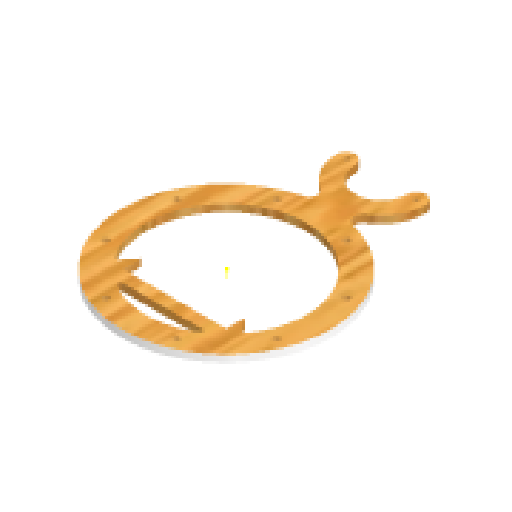
# Autodesk Inventor part: SparRing Curved
Saved by Autodesk Inventor 2025.2 (Build 292293000, 293)
## iProperties
Created: 2024-11-15
Part Number: SparRing Curved
Material: Plywood, Finish
Document SubType Name: Modeling
Designer: alexb
Density: 0.552 g/cm^3
Appearance: Plywood - New
Finish1_Area: 30458.089 mm^2
Finish1_Appearance: Plywood - New
Author: alexb
Autodesk Inventor part; units mm, degrees
ref_plane "YZ Plane" through (0, 0, 0) normal (1, 0, 0) x (0, 1, 0)
ref_plane "XZ Plane" through (0, 0, 0) normal (0, 1, 0) x (-1, 0, 0)
ref_plane "XY Plane" through (0, 0, 0) normal (0, 0, 1) x (1, 0, 0)
sketch "Sketch1" plane through (0, 0, 0) normal (0, 1, 0) x (-1, 0, 0)
  arc A0 (20, -82.6136) -> (-20, -82.6136) centre (0, 0) ccw
  line L0 (0, 0) -> (0, -85)
  line L1 (0, 0) -> (32.5281, -78.5298)
  circle A1 centre (0, 0) radius 75 construction
  circle A2 centre (28.7013, -69.291) radius 2.5
  line L2 (41, -41) -> (-41, -41) construction
  line L3 (-41, -41) -> (-41, 41) construction
  line L4 (-41, 41) -> (41, 41) construction
  line L5 (41, 41) -> (41, -41) construction
  line L6 (0, 0) -> (-85, 0)
  circle A3 centre (69.291, -28.7013) radius 2.5
  circle A4 centre (69.291, 28.7013) radius 2.5
  circle A5 centre (28.7013, 69.291) radius 2.5
  circle A6 centre (-28.7013, 69.291) radius 2.5
  circle A7 centre (-69.291, 28.7013) radius 2.5
  circle A8 centre (-69.291, -28.7013) radius 2.5
  circle A9 centre (-28.7013, -69.291) radius 2.5
  line L7 (42, 27) -> (42, 42)
  line L8 (42, 42) -> (-42, 42)
  line L9 (-42, 42) -> (-42, 27)
  line L10 (42, 27) -> (52.0326, 38.9564)
  line L11 (-39, 52) -> (39, 52)
  line L12 (-42, 27) -> (-52.0326, 38.9564)
  arc A10 (-52.0326, 38.9564) -> (52.0326, 38.9564) centre (0, 0) ccw
  arc A11 (39, 52) -> (-39, 52) centre (0, 0) ccw
  arc A12 (21, -126) -> (-21, -126) centre (0, -126) ccw
  line L13 (0, -105) -> (0, -85) construction
  arc A13 (-20, -82.6136) -> (20, -82.6136) centre (0, 0) ccw construction
  line L14 (0, -126) -> (36, -126) construction
  arc A14 (27.5132, -133.4348) -> (-27.5132, -133.4348) centre (0, -126) ccw
  circle A15 centre (28.5, -126) radius 2
  circle A16 centre (-28.5, -126) radius 2
  arc A17 (-20, -96.0667) -> (-36, -126) centre (0, -126) ccw
  arc A18 (36, -126) -> (20, -96.0667) centre (0, -126) ccw
  arc A19 (21, -126) -> (36, -126) centre (28.5, -126) ccw
  line L15 (0, -126) -> (-36, -126) construction
  arc A20 (-36, -126) -> (-21, -126) centre (-28.5, -126) ccw
  line L16 (-20, -89.3401) -> (-15, -89.3401) construction
  spline S0 degree 4 poles (-20, -82.6136) (-15.4558, -83.7137) (-12.0866, -90.2039) (-16.4143, -93.671) (-20, -96.0667) knots 0 0 0 0 0 1 1 1 1 1
  spline S1 degree 4 poles (20, -82.6136) (15.4558, -83.7137) (12.0866, -90.2039) (16.4143, -93.671) (20, -96.0667) knots 0 0 0 0 0 1 1 1 1 1
  line L17 (20, -89.3401) -> (15, -89.3401) construction
  line L18 (20, -96.0667) -> (20, -82.6136) construction
  line L19 (-20, -96.0667) -> (-20, -82.6136) construction
  point P0 (0, -41)
  point P1 (-41, 0)
  point P2 (0, 52)
  point P3 (17.5, -89.3401)
  dimension "d4" = 150
  dimension "d0" = 170
  dimension "d3" = 22.5
  dimension "d6" = 82
  dimension "d10" = 360
  dimension "d12" = 5
  dimension "d13" = 1
  dimension "d14" = 1
  dimension "d15" = 1
  dimension "d16" = 15
  dimension "d17" = 40
  dimension "d18" = 10
  dimension "d19" = 40
  dimension "d20" = 20
  dimension "d21" = 42
  dimension "d25" = 20
  dimension "d28" = 57
  dimension "d32" = 360
  dimension "d34" = 4
  dimension "d37" = 15
  dimension "d41" = 5
  dimension "d42" = 6.7266
  dimension "d43" = 6.7266
  dimension "d44" = 30
  constraints: 40 end point, 25 point on circle, 20 centre point, 8 coincident, 8 horizontal, 5 point on line, 5 vertical, 4 midpoint, 3 parallel, 3 perpendicular, 2 concentric, 2 equal length, 1 symmetric about line, 36 other
  measures "d0" diameter of A0
  measures "d3" angle of L0 L1
  measures "d6" distance of L2.start L2.end
  measures "d12" diameter of A9
  measures "d13" distance between parallel lines of L5 L7
  measures "d14" distance between parallel lines of L8 L4
  measures "d15" distance between parallel lines of L3 L9
  measures "d16" distance of L7.start L7.end
  measures "d17" angle of L10 L7
  measures "d18" distance from line of point (0, 52) L8
  measures "d19" angle of L9 L12
  measures "d20" radial gap between concentric circles of A0 A10
  measures "d21" diameter of A12
  measures "d25" distance of L13.start L0.end
  measures "d28" diameter of A14
  measures "d34" diameter of A16
  measures "d37" radial gap between concentric circles of A17 A12
  measures "d41" distance of L16.start L16.end
  measures "d42" vertical distance of L19.end L16.end
  measures "d43" vertical distance of L17.end A0.start
  measures "d44" distance of L16.end L17.end
extrude "Extrusion1" add sketch "Sketch1" along normal blind 6 contours S1 A18 A19 A14 A15 A16 A20 A17 S0 A0 L6 A10 L1 A2 | L1 A2 A10 L10 L7 L8 L9 L12 L6 A0 | A19 A12 A20 A14 A16 A15
sketch "Sketch2" plane through (0, 6, 0) normal (0, 1, 0) x (1, 0, 0)
  point P0 (0, 0)
fillet "Fillet1" radius 2 4 edges at (-39, 3, 52) (39, 3, 52) (-52.0326, 3, 38.9564) (52.0326, 3, 38.9564)
equation "\"d14\" = d13"
equation "\"d15\" = d13"
equation "\"d19\" = d17"
body "Solid1"
